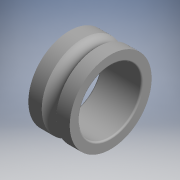
# Autodesk Inventor part: 673 Inner ring
Saved by Autodesk Inventor 2017.3 (Build 213256000, 256)
## iProperties
Part Number: 673 Inner ring
Material: Generic
Catalog Web Link: www.cadenas.de
Description: Six types ir-Metric system sizes
Vendor: NTN
Document SubType Name: Modeling
Designer: partserver
Manufacturer: NTN
Mass: 0.00944209 g
Surface Area: 0.543616 cm^2
Volume: 0.00944209 cm^3
Density: 1 g/cm^3
Appearance: PSOLRGB-192-192-192
Category: PARTsolutions
Company: NTN
Title: 673 Inner ring
Author: Cadenas PARTsolutions
Comments: Metric system sizes
PSOL_IDENT_0: {$CADENAS_DATA\23d-libs\ntn\ball_roller_bearings\miniature_extra_small_bb\metric_system_sizes\mss_ir
PSOL_IDENT_1: .prj},175 {VTYP=3D},{NB=673 Inner ring},{LINA=673 Inner ring},{NN=Six types ir},{DATE=21.12.2021 04:
PSOL_IDENT_2: 23:04},{GEOMDATE=06.03.2020 10:06:06},{VERSION=},{LINEID=450},{WBVAR=},{WBNUMERIC=}  {NB=673 Inner r
PSOL_IDENT_3: ing},{LINA=673 Inner ring},{KT=DUMMY},{IDNR=},{SD=3.0},{D=6},{B=2.0},{R=0.08},{ORDER=673},{CR=242},{
PSOL_IDENT_4: COR=94},{CRF=25},{CORF=9,5},{LSG=60 000},{LSO=71 000},{MASS=0.20},{D1=7.2},{D2=7.2},{C1=0.6},{C2=0.6
PSOL_IDENT_5: },{ORDER1=673},{WSS=WA673SA},{WDS=SSA},{UTWF=FL673},{FORSS=FLWA673SA},{FORDS=SSA},{DA1=3,6},{DA2=4,1
PSOL_IDENT_6: },{DA=5,4},{RAS=0,08},{MASS1=0.26},{B1=2.5},{VERS=1},{X=1.5},{N=9},{O=14.13},{RB=0.444}
NB: 673 Inner ring
NN: Six types ir
NT: Metric system sizes
NBSYN: $ORDER. Inner ring
LINA: 673 Inner ring
CATALOG: NTN Corporation
SD: 3
D: 6
B: 2
R: 0.08
CR: 242
COR: 94
CRF: 25
CORF: 9,5
LSG: 60 000
LSO: 71 000
MASS: 0.2
D1: 7.2
D2: 7.2
C1: 0.6
C2: 0.6
ORDER1: 673
WSS: WA673SA
WDS: SSA
UTWF: FL673
FORSS: FLWA673SA
FORDS: SSA
DA1: 3,6
DA2: 4,1
DA: 5,4
RAS: 0,08
MASS1: 0.26
B1: 2.5
VERS: 1
SUPPLIER: NTN
ARTICLENO: 673 Inner ring
BOMINFO: 673 Inner ring
CREATOR: CADENAS GmbH
Autodesk Inventor part; units mm, degrees
sketch "Sketch_1" plane through (0, 0, 0) normal (0, 0, 1) x (1, 0, 0)
  line L0 (2, 0) -> (0, 0)
  arc A0 (0, 1.58) -> (0.08, 1.5) centre (0.08, 1.58) ccw
  line L1 (0.08, 1.5) -> (1.92, 1.5)
  arc A1 (1.92, 1.5) -> (2, 1.58) centre (1.92, 1.58) ccw
  line L2 (2, 1.58) -> (2, 1.98)
  line L3 (2, 1.98) -> (1.3525, 1.98)
  arc A2 (0.6475, 1.98) -> (1.3525, 1.98) centre (1, 2.25) ccw
  line L4 (0.6475, 1.98) -> (0, 1.98)
  line L5 (0, 1.98) -> (0, 1.58)
  constraints: 12 end point, 6 point on circle, 3 centre point
revolve "Revolution1" add sketch "Sketch_1" angle 360 about axis through (2, 0, 0) along (1, 0, 0)
ref_plane "mss_ir_XY" through (0, 0, 0) normal (1, 0, 0) x (0, 0, -1)
ref_plane "mss_ir_YZ" through (0, 0, 0) normal (0, 0, -1) x (0, 1, 0)
ref_plane "mss_ir_ZX" through (0, 0, 0) normal (0, 1, 0) x (1, 0, 0)
body "Solid1"
